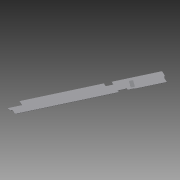
# Autodesk Inventor part: LabVIEWM0.5
Saved by Autodesk Inventor 2013 SP2 (Build 170200200, 200)
## iProperties
Created: 2014-11-17
Part Number: LabVIEWM0.5
Material: 常规
Document SubType Name: Modeling
Designer: 振胜
Density: 1 g/cm^3
Author: 振胜
Autodesk Inventor part; units mm, degrees
ref_plane "YZ Plane" through (0, 0, 0) normal (1, 0, 0) x (0, 1, 0)
sketch "DOOR" plane through (0, 0, 0) normal (0, 0, 1) x (1, 0, 0)
  line L0 (-118.2333, 89.8968) -> (-138.2333, 89.8968)
  line L1 (-138.2333, 89.8968) -> (-138.2333, 79.8968)
  line L2 (-138.2333, 79.8968) -> (-118.2333, 79.8968)
  line L3 (-118.2333, 79.8968) -> (-118.2333, 89.8968)
  line L4 (-118.2333, 84.8968) -> (-138.2333, 84.8968) construction
  dimension "d362" = 10
  dimension "d364" = 20
  measures "d362" distance of L0.end L1.end
  measures "d364" distance of L0.start L0.end
sketch "DOOR2" plane through (0, 0, 0) normal (0, 0, 1) x (1, 0, 0)
  line L0 (127.9548, -63.9092) -> (147.9548, -63.9092)
  line L1 (147.9548, -63.9092) -> (147.9548, -73.9092)
  line L2 (147.9548, -73.9092) -> (127.9548, -73.9092)
  line L3 (127.9548, -73.9092) -> (127.9548, -63.9092)
  line L4 (127.9548, -68.9092) -> (147.9548, -68.9092) construction
  dimension "d382" = 10
  dimension "d384" = 20
  measures "d382" distance of L0.end L1.end
  measures "d384" distance of L0.start L0.end
ref_plane "工作平面1" through (0, 0, 15) normal (0, 0, 1) x (1, 0, 0)
sketch "草图1" plane through (0, 0, 15) normal (0, 0, 1) x (1, 0, 0)
  line L0 (849.2, -1174.6) -> (1031.2, -1174.6)
  line L1 (1031.2, -1121.1) -> (909.2, -1121.1)
  line L2 (1031.2, -1121.1) -> (1031.2, -1174.6)
  line L3 (916.6396, -626.805) -> (1226.8396, -727.205) construction
  arc A0 (1226.8396, -727.205) -> (916.6396, -626.805) centre (762.4326, -1632.6529) ccw
  line L4 (916.6396, -664.805) -> (1213.8396, -757.905) construction
  arc A1 (1213.8396, -757.905) -> (916.6396, -664.805) centre (606.0403, -2177.2415) ccw
  line L5 (1226.8396, -727.205) -> (1213.8396, -757.905)
  line L6 (1226.8396, -727.205) -> (1240.1864, -734.0506)
  line L7 (1213.8396, -757.905) -> (1227.1864, -764.7506)
  line L8 (1240.1864, -734.0506) -> (1237.5395, -739.2114)
  line L9 (1227.1864, -764.7506) -> (1224.5874, -769.8179)
  line L10 (1031.2, -1121.1) -> (1046.2, -1121.1)
  line L11 (1046.2, -1121.1) -> (1046.2, -1174.6)
  line L12 (1046.2, -1174.6) -> (1031.2, -1174.6)
  line L13 (1046.2, -1121.1) -> (1068.2, -1121.1)
  line L14 (1068.2, -1174.6) -> (1046.2, -1174.6)
  line L15 (1068.2, -1121.1) -> (1068.2, -1139.5)
  line L16 (1068.2, -1174.6) -> (1068.2, -1156.2)
  line L17 (1068.2, -1174.6) -> (1110, -1180.4746)
  line L18 (1068.2, -1121.1) -> (1117.8, -1121.1)
  line L19 (1110, -1180.4746) -> (1113.8458, -1172.2272)
  line L20 (1113.8458, -1172.2272) -> (1141.0351, -1184.9058)
  line L21 (1141.0351, -1184.9058) -> (1162.5041, -1138.8653)
  line L22 (1162.5041, -1138.8653) -> (1176.9999, -1107.779)
  line L23 (1176.9999, -1107.779) -> (1192.5945, -1074.3362)
  line L24 (1192.5945, -1074.3362) -> (1207.7242, -1041.8904)
  line L25 (1207.7242, -1041.8904) -> (1223.0653, -1008.9914)
  line L26 (1223.0653, -1008.9914) -> (1238.4063, -976.0924)
  line L27 (1238.4063, -976.0924) -> (1261.439, -926.6987)
  line L28 (1261.439, -926.6987) -> (1283.7532, -878.8456)
  line L29 (1283.7532, -878.8456) -> (1305.8562, -831.4457)
  line L30 (1305.8562, -831.4457) -> (1329.8609, -779.9674)
  line L31 (1117.8, -1121.1) -> (1090.6108, -1108.4215)
  line L32 (1090.6108, -1108.4215) -> (1107.8959, -1071.3535)
  line L33 (1107.8959, -1071.3535) -> (1122.3494, -1040.3577)
  line L34 (1122.3494, -1040.3577) -> (1135.4506, -1012.2622)
  line L35 (1135.4506, -1012.2622) -> (1150.6648, -979.6351)
  line L36 (1150.6648, -979.6351) -> (1170.2743, -937.5824)
  line L37 (1170.2743, -937.5824) -> (1183.1219, -910.0307)
  line L38 (1183.1219, -910.0307) -> (1198.4207, -877.2223)
  line L39 (1198.4207, -877.2223) -> (1213.6349, -844.5953)
  line L40 (1213.6349, -844.5953) -> (1224.7498, -820.7594)
  line L41 (1224.7498, -820.7594) -> (1244.2325, -778.9786)
  line L42 (1224.5874, -769.8179) -> (1271.7154, -791.7941)
  line L43 (1237.5395, -739.2114) -> (1285.7517, -761.6931)
  line L44 (1271.7154, -791.7941) -> (1285.7517, -761.6931) construction
  line L45 (1244.2325, -778.9786) -> (1258.2688, -748.8776) construction
  line L46 (1258.2688, -748.8776) -> (1274.4973, -714.0754)
  line L47 (1274.4973, -714.0754) -> (1289.458, -681.9921)
  line L48 (1289.458, -681.9921) -> (1304.2497, -650.2714)
  line L49 (1304.2497, -650.2714) -> (1321.3657, -613.5659)
  line L50 (1321.3657, -613.5659) -> (1325.0425, -605.681)
  line L51 (1325.0425, -605.681) -> (1350.1883, -551.7557)
  line L52 (1350.1883, -551.7557) -> (1377.3775, -564.4342)
  line L53 (1377.3775, -564.4342) -> (1390.1051, -579.0756)
  line L54 (1390.1051, -579.0756) -> (1417.2943, -591.7542)
  line L55 (1377.3775, -564.4342) -> (1350.1883, -551.7557)
  line L56 (1350.1883, -551.7557) -> (1325.0425, -605.681)
  line L57 (1325.0425, -605.681) -> (1352.2317, -618.3596)
  line L58 (1352.2317, -618.3596) -> (1377.3775, -564.4342)
  line L59 (1352.2317, -618.3596) -> (1325.0425, -605.681)
  line L60 (1325.0425, -605.681) -> (1304.2497, -650.2714)
  line L61 (1304.2497, -650.2714) -> (1331.4389, -662.9499)
  line L62 (1331.4389, -662.9499) -> (1352.2317, -618.3596)
  line L63 (1331.4389, -662.9499) -> (1304.2497, -650.2714)
  line L64 (1304.2497, -650.2714) -> (1289.458, -681.9921)
  line L65 (1289.458, -681.9921) -> (1316.6473, -694.6707)
  line L66 (1316.6473, -694.6707) -> (1331.4389, -662.9499)
  line L67 (1316.6473, -694.6707) -> (1289.458, -681.9921)
  line L68 (1289.458, -681.9921) -> (1274.4973, -714.0754)
  line L69 (1274.4973, -714.0754) -> (1301.6866, -726.754)
  line L70 (1301.6866, -726.754) -> (1316.6473, -694.6707)
  line L71 (1301.6866, -726.754) -> (1274.4973, -714.0754)
  line L72 (1274.4973, -714.0754) -> (1258.2688, -748.8776)
  line L73 (1258.2688, -748.8776) -> (1285.458, -761.5562)
  line L74 (1285.458, -761.5562) -> (1301.6866, -726.754)
  line L75 (1417.2943, -591.7542) -> (1406.3907, -615.1369)
  line L76 (1406.3907, -615.1369) -> (1395.4872, -638.5196)
  line L77 (1395.4872, -638.5196) -> (1391.8104, -646.4045)
  line L78 (1391.8104, -646.4045) -> (1375.1592, -682.113)
  line L79 (1375.1592, -682.113) -> (1357.7474, -719.4529)
  line L80 (1390.1051, -579.0756) -> (1417.2943, -591.7542)
  line L81 (1417.2943, -591.7542) -> (1406.3907, -615.1369)
  line L82 (1406.3907, -615.1369) -> (1379.2015, -602.4583)
  line L83 (1379.2015, -602.4583) -> (1390.1051, -579.0756)
  line L84 (1379.2015, -602.4583) -> (1406.3907, -615.1369)
  line L85 (1406.3907, -615.1369) -> (1395.4872, -638.5196)
  line L86 (1395.4872, -638.5196) -> (1368.2979, -625.8411)
  line L87 (1368.2979, -625.8411) -> (1379.2015, -602.4583)
  line L88 (1368.2979, -625.8411) -> (1395.4872, -638.5196)
  line L89 (1395.4872, -638.5196) -> (1391.8104, -646.4045)
  line L90 (1391.8104, -646.4045) -> (1364.6212, -633.726)
  line L91 (1364.6212, -633.726) -> (1368.2979, -625.8411)
  line L92 (1364.6212, -633.726) -> (1391.8104, -646.4045)
  line L93 (1391.8104, -646.4045) -> (1375.1592, -682.113)
  line L94 (1375.1592, -682.113) -> (1347.97, -669.4345)
  line L95 (1347.97, -669.4345) -> (1364.6212, -633.726)
  line L96 (1347.97, -669.4345) -> (1375.1592, -682.113)
  line L97 (1375.1592, -682.113) -> (1357.7474, -719.4529)
  line L98 (1357.7474, -719.4529) -> (1330.5581, -706.7744)
  line L99 (1330.5581, -706.7744) -> (1347.97, -669.4345)
  line L100 (1330.5581, -706.7744) -> (1345.9654, -713.9589)
  line L101 (1345.9654, -713.9589) -> (1331.1737, -745.6797)
  line L102 (1331.1737, -745.6797) -> (1315.7665, -738.4951)
  line L103 (1315.7665, -738.4951) -> (1330.5581, -706.7744)
  line L104 (1113.8458, -1172.2272) -> (1141.0351, -1184.9058)
  line L105 (1141.0351, -1184.9058) -> (1162.5041, -1138.8653)
  line L106 (1162.5041, -1138.8653) -> (1135.3148, -1126.1868)
  line L107 (1135.3148, -1126.1868) -> (1113.8458, -1172.2272)
  line L108 (1135.3148, -1126.1868) -> (1162.5041, -1138.8653)
  line L109 (1162.5041, -1138.8653) -> (1176.9999, -1107.779)
  line L110 (1176.9999, -1107.779) -> (1149.8106, -1095.1004)
  line L111 (1149.8106, -1095.1004) -> (1135.3148, -1126.1868)
  line L112 (1149.8106, -1095.1004) -> (1176.9999, -1107.779)
  line L113 (1176.9999, -1107.779) -> (1192.5945, -1074.3362)
  line L114 (1192.5945, -1074.3362) -> (1165.4053, -1061.6577)
  line L115 (1165.4053, -1061.6577) -> (1149.8106, -1095.1004)
  line L116 (1165.4053, -1061.6577) -> (1192.5945, -1074.3362)
  line L117 (1192.5945, -1074.3362) -> (1207.7242, -1041.8904)
  line L118 (1207.7242, -1041.8904) -> (1180.535, -1029.2118)
  line L119 (1180.535, -1029.2118) -> (1165.4053, -1061.6577)
  line L120 (1180.535, -1029.2118) -> (1207.7242, -1041.8904)
  line L121 (1207.7242, -1041.8904) -> (1223.0653, -1008.9914)
  line L122 (1223.0653, -1008.9914) -> (1195.876, -996.3129)
  line L123 (1195.876, -996.3129) -> (1180.535, -1029.2118)
  line L124 (1195.876, -996.3129) -> (1223.0653, -1008.9914)
  line L125 (1223.0653, -1008.9914) -> (1238.4063, -976.0924)
  line L126 (1238.4063, -976.0924) -> (1211.2171, -963.4139)
  line L127 (1211.2171, -963.4139) -> (1195.876, -996.3129)
  line L128 (1211.2171, -963.4139) -> (1238.4063, -976.0924)
  line L129 (1238.4063, -976.0924) -> (1261.439, -926.6987)
  line L130 (1261.439, -926.6987) -> (1234.2498, -914.0201)
  line L131 (1234.2498, -914.0201) -> (1211.2171, -963.4139)
  line L132 (1234.2498, -914.0201) -> (1261.439, -926.6987)
  line L133 (1261.439, -926.6987) -> (1283.7532, -878.8456)
  line L134 (1283.7532, -878.8456) -> (1256.564, -866.1671)
  line L135 (1256.564, -866.1671) -> (1234.2498, -914.0201)
  line L136 (1256.564, -866.1671) -> (1283.7532, -878.8456)
  line L137 (1283.7532, -878.8456) -> (1305.8562, -831.4457)
  line L138 (1305.8562, -831.4457) -> (1278.6669, -818.7672)
  line L139 (1278.6669, -818.7672) -> (1256.564, -866.1671)
  line L140 (1278.6669, -818.7672) -> (1305.8562, -831.4457)
  line L141 (1305.8562, -831.4457) -> (1329.9336, -779.8115)
  line L142 (1329.9336, -779.8115) -> (1302.7444, -767.1329)
  line L143 (1302.7444, -767.1329) -> (1278.6669, -818.7672)
  line L144 (1117.8, -1121.1) -> (1090.6108, -1108.4215)
  line L145 (1090.6108, -1108.4215) -> (1107.8959, -1071.3535)
  line L146 (1107.8959, -1071.3535) -> (1135.0851, -1084.032)
  line L147 (1135.0851, -1084.032) -> (1117.8, -1121.1)
  line L148 (1135.0851, -1084.032) -> (1107.8959, -1071.3535)
  line L149 (1107.8959, -1071.3535) -> (1122.3494, -1040.3577)
  line L150 (1122.3494, -1040.3577) -> (1149.5386, -1053.0363)
  line L151 (1149.5386, -1053.0363) -> (1135.0851, -1084.032)
  line L152 (1149.5386, -1053.0363) -> (1122.3494, -1040.3577)
  line L153 (1122.3494, -1040.3577) -> (1135.4506, -1012.2622)
  line L154 (1135.4506, -1012.2622) -> (1162.6398, -1024.9407)
  line L155 (1162.6398, -1024.9407) -> (1149.5386, -1053.0363)
  line L156 (1162.6398, -1024.9407) -> (1135.4506, -1012.2622)
  line L157 (1135.4506, -1012.2622) -> (1150.6648, -979.6351)
  line L158 (1150.6648, -979.6351) -> (1177.8541, -992.3137)
  line L159 (1177.8541, -992.3137) -> (1162.6398, -1024.9407)
  line L160 (1177.8541, -992.3137) -> (1150.6648, -979.6351)
  line L161 (1150.6648, -979.6351) -> (1170.2743, -937.5824)
  line L162 (1170.2743, -937.5824) -> (1197.4635, -950.261)
  line L163 (1197.4635, -950.261) -> (1177.8541, -992.3137)
  line L164 (1197.4635, -950.261) -> (1170.2743, -937.5824)
  line L165 (1170.2743, -937.5824) -> (1183.1219, -910.0307)
  line L166 (1183.1219, -910.0307) -> (1210.3111, -922.7092)
  line L167 (1210.3111, -922.7092) -> (1197.4635, -950.261)
  line L168 (1210.3111, -922.7092) -> (1183.1219, -910.0307)
  line L169 (1183.1219, -910.0307) -> (1198.4207, -877.2223)
  line L170 (1198.4207, -877.2223) -> (1225.6099, -889.9009)
  line L171 (1225.6099, -889.9009) -> (1210.3111, -922.7092)
  line L172 (1225.6099, -889.9009) -> (1198.4207, -877.2223)
  line L173 (1198.4207, -877.2223) -> (1213.6349, -844.5953)
  line L174 (1213.6349, -844.5953) -> (1240.8242, -857.2738)
  line L175 (1240.8242, -857.2738) -> (1225.6099, -889.9009)
  line L176 (1240.8242, -857.2738) -> (1213.6349, -844.5953)
  line L177 (1213.6349, -844.5953) -> (1224.7498, -820.7594)
  line L178 (1224.7498, -820.7594) -> (1251.939, -833.4379)
  line L179 (1251.939, -833.4379) -> (1240.8242, -857.2738)
  line L180 (1251.939, -833.4379) -> (1224.7498, -820.7594)
  line L181 (1224.7498, -820.7594) -> (1249.6843, -767.2872)
  line L182 (1249.6843, -767.2872) -> (1276.8735, -779.9657)
  line L183 (1276.8735, -779.9657) -> (1251.939, -833.4379)
  line L184 (1331.1737, -745.6797) -> (1332.08, -746.1023)
  line L185 (1332.08, -746.1023) -> (1318.7853, -774.6129)
  line L186 (1302.7444, -767.1329) -> (1315.7665, -738.4951) construction
  point P0 (0, 0)
  dimension "d122" = 182
  dimension "d123" = 100.4
  dimension "d124" = 310.2
  dimension "d125" = 1017.6
  dimension "d126" = 93.1
  dimension "d127" = 297.2
  dimension "d128" = 1544
  dimension "d129" = 15
  dimension "d130" = 15
  dimension "d131" = 5.8
  dimension "d133" = 15
  dimension "d134" = 22
  dimension "d135" = 18.4
  dimension "d136" = 18.4
  dimension "d137" = 172
  dimension "d138" = 41.8
  dimension "d139" = 49.6
  dimension "d140" = 107
  dimension "d141" = 9.1
  dimension "d142" = 30
  dimension "d143" = 50.8
  dimension "d144" = 34.3
  dimension "d145" = 36.9
  dimension "d146" = 35.8
  dimension "d147" = 36.3
  dimension "d148" = 36.3
  dimension "d149" = 54.5
  dimension "d150" = 52.8
  dimension "d151" = 52.3
  dimension "d152" = 56.8
  dimension "d153" = 30
  dimension "d154" = 40.9
  dimension "d155" = 34.2
  dimension "d156" = 31
  dimension "d157" = 36
  dimension "d158" = 46.4
  dimension "d159" = 30.4
  dimension "d160" = 36.2
  dimension "d161" = 36
  dimension "d162" = 26.3
  dimension "d163" = 46.1
  dimension "d164" = 52
  dimension "d165" = 38.4
  dimension "d166" = 35.4
  dimension "d167" = 35
  dimension "d168" = 40.5
  dimension "d169" = 8.7
  dimension "d170" = 59.5
  dimension "d171" = 30
  dimension "d172" = 156
  dimension "d173" = 19.4
  dimension "d174" = 30
  dimension "d175" = 25.8
  dimension "d176" = 25.8
  dimension "d177" = 8.7
  dimension "d178" = 39.4
  dimension "d179" = 41.2
  dimension "d180" = 17
  dimension "d181" = 35
  dimension "d183" = 1
  dimension "d184" = 0.548
  dimension "d185" = 87.95
  dimension "d186" = 25
  dimension "d187" = 25
  constraints: 376 end point, 73 parallel, 59 perpendicular, 43 collinear, 5 point on line, 4 point on circle, 2 centre point, 1 tangent, 1 vertical
  measures "d122" distance of L0.start L0.end
  measures "d123" vertical distance of L3.start L3.end
  measures "d124" horizontal distance of L3.end L3.start
  measures "d125" radius of A0
  measures "d126" vertical distance of L4.end L4.start
  measures "d127" horizontal distance of L4.end L4.start
  measures "d128" radius of A1
  measures "d129" distance of L3.end L6.end
  measures "d130" distance of L4.end L7.end
  measures "d131" distance of L6.end L8.end
  measures "d133" distance of L1.start L10.end
  measures "d134" distance of L10.end L13.end
  measures "d135" distance of L13.end L15.end
  measures "d136" distance of L14.start L16.end
  measures "d137" angle of L17 L14
  measures "d138" horizontal distance of L17.end L14.start
  measures "d139" distance of L13.end L18.end
  measures "d140" angle of L17 L19
  measures "d141" distance of L17.end L19.end
  measures "d142" distance of L19.end L20.end
  measures "d143" distance of L20.end L21.end
  measures "d144" distance of L21.end L22.end
  measures "d145" distance of L22.end L23.end
  measures "d146" distance of L23.end L24.end
  measures "d147" distance of L24.end L25.end
  measures "d148" distance of L25.end L26.end
  measures "d149" distance of L26.end L27.end
  measures "d150" distance of L27.end L28.end
  measures "d151" distance of L28.end L29.end
  measures "d152" distance of L29.end L30.end
  measures "d153" distance of L18.end L31.end
  measures "d154" distance of L31.end L32.end
  measures "d155" distance of L32.end L33.end
  measures "d156" distance of L33.end L34.end
  measures "d157" distance of L34.end L35.end
  measures "d158" distance of L35.end L36.end
  measures "d159" distance of L36.end L37.end
  measures "d160" distance of L37.end L38.end
  measures "d161" distance of L38.end L39.end
  measures "d162" distance of L39.end L40.end
  measures "d163" distance of L40.end L41.end
  measures "d164" distance of L9.end L42.end
  measures "d165" distance of L45.end L46.end
  measures "d166" distance of L46.end L47.end
  measures "d167" distance of L47.end L48.end
  measures "d168" distance of L48.end L49.end
  measures "d169" distance of L49.end L50.end
  measures "d170" distance of L50.end L51.end
  measures "d171" distance of L51.end L52.end
  measures "d172" angle of L53 L52
  measures "d173" distance of L52.end L53.end
  measures "d174" distance of L53.end L54.end
  measures "d175" distance of L54.end L75.end
  measures "d176" distance of L75.end L76.end
  measures "d177" distance of L76.end L77.end
  measures "d178" distance of L77.end L78.end
  measures "d179" distance of L78.end L79.end
  measures "d180" distance of L98.end L100.end
  measures "d181" distance of L100.end L101.end
  measures "d183" distance of L101.end L184.end
  measures "d184" angle of L75 L186
  measures "d185" angle of L54 L5
  measures "d186" angle of L54 L1
  measures "d187" angle of L54 L0
extrude "拉伸5" add sketch "草图1" against normal blind 1
sketch "草图6" plane through (0, 0, 15) normal (0, 0, 1) x (1, 0, 0)
  line L0 (1350.1883, -551.7557) -> (1258.2688, -748.8776) construction
  line L1 (1244.2325, -778.9786) -> (1090.6108, -1108.4215) construction
  line L2 (1258.2688, -748.8776) -> (1237.5395, -739.2114) construction
  line L3 (1224.5874, -769.8179) -> (1244.2325, -778.9786) construction
  line L4 (1258.2688, -748.8776) -> (1250.0214, -745.0318) construction
  line L5 (1250.0214, -745.0318) -> (1235.9851, -775.1327)
  line L6 (1235.9851, -775.1327) -> (1244.2325, -778.9786) construction
  line L7 (1250.0214, -745.0318) -> (1277.2106, -757.7104)
  line L8 (1235.9851, -775.1327) -> (1263.1743, -787.8113)
  line L9 (1263.1743, -787.8113) -> (1277.2106, -757.7104)
  line L10 (1237.5395, -739.2114) -> (1240.1864, -734.0506) construction
  line L11 (1240.1864, -734.0506) -> (1226.8396, -727.205) construction
  line L12 (1213.8396, -757.905) -> (1227.1864, -764.7506) construction
  line L13 (1227.1864, -764.7506) -> (1224.5874, -769.8179) construction
  line L14 (1226.8396, -727.205) -> (1213.8396, -757.905) construction
  line L15 (1250.0214, -745.0318) -> (1237.5395, -739.2114)
  line L16 (1237.5395, -739.2114) -> (1240.1864, -734.0506)
  line L17 (1240.1864, -734.0506) -> (1226.8396, -727.205)
  line L18 (1226.8396, -727.205) -> (1213.8396, -757.905)
  line L19 (1213.8396, -757.905) -> (1227.1864, -764.7506)
  line L20 (1227.1864, -764.7506) -> (1224.5874, -769.8179)
  line L21 (1224.5874, -769.8179) -> (1235.9851, -775.1327)
  point P0 (0, 0)
  dimension "d411" = 9.1
  dimension "d412" = 30
  dimension "d413" = 30
  constraints: 26 end point, 6 collinear, 3 point on line, 2 perpendicular, 1 parallel
  measures "d411" distance of L0.end L4.end
  measures "d412" distance of L4.end L7.end
  measures "d413" distance of L5.end L8.end
extrude "拉伸6" cut sketch "草图6" against normal blind 10
ref_plane "工作平面2" through (1338.5696, -729.8193, 14) normal (-0.4226183, -0.9063078, 0) x (0.9063078, -0.4226183, 0)
sketch "草图7" plane through (1338.5696, -729.8193, 14) normal (-0.4226183, -0.9063078, 0) x (0.9063078, -0.4226183, 0)
  line L0 (0, 1) -> (0, 0) construction
  line L1 (0, 0.5) -> (22.5, 17.75)
  line L2 (22.5, 18.15) -> (22.5, 17.75)
  line L3 (22.5, 18.15) -> (32.5, 18.15)
  line L4 (32.5, 18.15) -> (32.5, 17.75)
  line L5 (0, 0.5) -> (0, 0.9)
  line L6 (0, 0.9) -> (22.5, 18.15)
  line L7 (32.5, 17.75) -> (22.5, 17.75)
  point P0 (-1521.591, -14)
  dimension "d416" = 17.25
  dimension "d418" = 22.5
  dimension "d419" = 10
  dimension "d420" = 0.4
  constraints: 14 end point, 2 parallel, 2 perpendicular, 1 midpoint, 1 point on line, 1 vertical
  measures "d416" vertical distance of L1.start L1.end
  measures "d418" horizontal distance of L1.start L1.end
  measures "d419" distance of L2.start L3.end
  measures "d420" distance of L1.start L5.end
extrude "拉伸7" add sketch "草图7" along normal up to surface (17.5 mm away)
sketch "草图8" plane through (1338.5696, -729.8193, 14) normal (0.4226183, 0.9063078, 0) x (0.9063078, -0.4226183, 0)
  line L0 (32.5, -17.75) -> (32.5, -18.15) construction
  line L1 (32.5, -18.15) -> (22.5, -18.15) construction
  line L2 (22.5, -17.75) -> (32.5, -17.75) construction
  line L3 (32.5, -18.15) -> (22.5, -18.15)
  line L4 (22.5, -18.15) -> (22.5, -17.75)
  line L5 (22.5, -17.75) -> (32.5, -17.75)
  line L6 (32.5, -17.75) -> (32.5, -18.15)
  line L7 (22.5, -17.75) -> (0, -35)
  line L8 (22.5, -18.15) -> (0, -35.4)
  line L9 (0, -35.4) -> (0, -35)
  point P0 (-1521.591, 14)
  dimension "d423" = 17.25
  dimension "d424" = 22.5
  constraints: 14 end point, 3 parallel, 1 horizontal, 1 perpendicular, 1 vertical
  measures "d423" vertical distance of L2.start L7.end
  measures "d424" horizontal distance of L2.start L7.end
extrude "拉伸8" add sketch "草图8" along normal up to surface (17.5 mm away)
sketch "草图9" plane through (0, 0, 15) normal (0, 0, 1) x (1, 0, 0)
  line L0 (1031.2, -1121.1) -> (1031.2, -1174.6) construction
  line L1 (1117.8, -1121.1) -> (1031.2, -1121.1) construction
  line L2 (1031.2, -1174.6) -> (1068.2, -1174.6) construction
  line L3 (1068.2, -1174.6) -> (1110, -1180.4746) construction
  line L4 (1110, -1180.4746) -> (1113.8458, -1172.2272) construction
  line L5 (1117.8, -1121.1) -> (1031.2, -1121.1)
  line L6 (1031.2, -1121.1) -> (1031.2, -1174.6)
  line L7 (1031.2, -1174.6) -> (1068.2, -1174.6)
  line L8 (1068.2, -1174.6) -> (1110, -1180.4746) construction
  line L9 (1110, -1180.4746) -> (1113.8458, -1172.2272) construction
  line L10 (1090.6108, -1108.4215) -> (1117.8, -1121.1) construction
  line L11 (1117.8, -1121.1) -> (1090.6108, -1108.4215) construction
  line L12 (1117.8, -1121.1) -> (1091.3363, -1177.8516)
  line L13 (1091.3363, -1177.8516) -> (1068.2, -1174.6)
  point P0 (0, 0)
  constraints: 16 end point, 7 collinear, 1 perpendicular, 1 point on line
extrude "拉伸9" cut sketch "草图9" against normal blind 10
